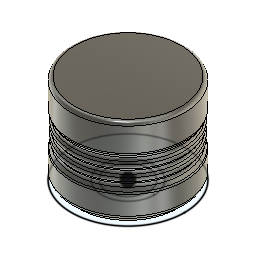
Soft Hammer Head v2 (Autodesk Fusion 360 design; units mm, degrees)
Autodesk Fusion 360 part; units mm, degrees
sketch "Sketch1" plane through (0, 0, 0) normal (0, 0, 1) x (1, 0, 0)
  circle A0 centre (0, 0) radius 16
  circle A1 centre (0, 0) radius 5.75
  circle A2 centre (0, 0) radius 7.375
  dimension "d7" = 32
  dimension "d8" = 11.5
  dimension "d9" = 14.75
  constraint coincident A0.centre A1.centre
  measures "d7" diameter of A0
  measures "d8" diameter of A1
  measures "d9" diameter of A2
extrude "Extrude1" add sketch "Sketch1" along normal blind 8 contours A0 | A1 | A2
extrude "Extrude2" add 1 faces at (3.3126, -0.5422, 8) along direction (0, 0, 1) blind 1.5833 draft -30
extrude "Extrude3" add 1 faces at (4.1548, -2.8327, 9.5833) along direction (0, 0, 1) blind 1.5833 draft 30
extrude "Extrude4" add 1 faces at (3.3126, -0.5422, 11.1667) along direction (0, 0, 1) blind 1.5833 draft -30
extrude "Extrude5" add 1 faces at (4.1548, -2.8327, 12.75) along direction (0, 0, 1) blind 1.5833 draft 30
extrude "Extrude6" add 1 faces at (-4.6978, -3.7464, 14.3333) along direction (0, 0, 1) blind 1.5833 draft -30
extrude "Extrude7" add 1 faces at (-7.4207, -2.8415, 15.9167) along direction (0, 0, 1) blind 1.5833 draft 30
extrude "Extrude8" add 1 faces at (-4.6978, -3.7464, 17.5) along direction (0, 0, 1) blind 8
extrude "Extrude9" cut sketch "Sketch1" along normal blind 14.1 contours A1
extrude "Extrude10" cut sketch "Sketch1" along normal blind 12.1 from surface at 2 contours A1 | A2
chamfer "Chamfer1" distance 1.625 angle 45 1 edges at (-5.3609, -2.0793, 2)
chamfer "Chamfer2" distance 1 angle 45 1 edges at (-6.8759, -2.6669, 14.1)
chamfer "Chamfer2" distance 2 angle 45 1 edges at (-14.9172, -5.7858, 0)
fillet "Fillet1" radius 1 9 edges at (-14.9172, 5.7858, 14.3333) (-14.9172, 5.7858, 11.1667) (-14.065, 5.4553, 12.75) (-14.065, 5.4553, 15.9167) (-14.9172, 5.7858, 17.5) (-14.065, 5.4553, 9.5833) (-14.9172, -5.7858, 8) (-14.9172, 5.7858, 2) (-14.9172, -5.7858, 25.5)
equation "id = 11.5 mm"
equation "od = 32 mm"
equation "notchwidth = 14.75 mm"
equation "pegDepth = 10.1 mm"
equation "ridgeStart = 8 mm"
equation "ridgeHeight = 9.5 mm"
equation "d7 = od"
equation "d8 = id"
equation "d9 = notchwidth"
equation "d10 = ridgeStart"
equation "d12 = ridgeHeight / 6"
equation "d13 = -ridgeAngle"
equation "d14 = ridgeHeight / ridgeCount"
equation "d15 = ridgeAngle"
equation "ridgeCount = 6"
equation "ridgeAngle = 30 deg"
equation "d18 = ridgeHeight / ridgeCount"
equation "d19 = -ridgeAngle"
equation "d20 = ridgeHeight / ridgeCount"
equation "d21 = ridgeAngle"
equation "d22 = ridgeHeight / ridgeCount"
equation "d23 = -ridgeAngle"
equation "d24 = ridgeHeight / ridgeCount"
equation "d25 = ridgeAngle"
equation "d26 = ridgeStart"
equation "d28 = pegDepth + 4 mm"
equation "d31 = pegDepth + 2 mm"
equation "d33 = ( notchwidth - id ) / 2"
